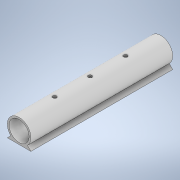
# Autodesk Inventor part: Cylinder
Saved by Autodesk Inventor 2022 (Build 260153000, 153)
## iProperties
Created: 2022-02-25
Part Number: Cylinder
Material: Generic
Document SubType Name: Modeling
Designer: Alexa
Density: 1 g/cm^3
Appearance: Default
Author: Alexa
Autodesk Inventor part; units mm, degrees
ref_plane "YZ Plane" through (0, 0, 0) normal (1, 0, 0) x (0, 1, 0)
ref_plane "XZ Plane" through (0, 0, 0) normal (0, 1, 0) x (-1, 0, 0)
ref_plane "XY Plane" through (0, 0, 0) normal (0, 0, 1) x (1, 0, 0)
sketch "Sketch1" plane through (0, 0, 0) normal (0, 1, 0) x (-1, 0, 0)
  line L0 (0, 0) -> (20, 0)
  line L1 (20, 0) -> (20, -120)
  line L2 (20, -120) -> (0, -120)
  line L3 (0, -120) -> (0, 0)
  dimension "d0" = 20
  dimension "d1" = 120
  constraints: 8 end point, 2 parallel, 1 horizontal, 1 perpendicular
  measures "d0" distance of L1.end L2.end
  measures "d1" distance of L0.end L1.end
extrude "Extrusion1" add sketch "Sketch1" along normal blind 20
sketch "Sketch2" plane through (0, 20, 0) normal (0, 1, 0) x (1, 0, 0)
  line L0 (-20, 120) -> (-20, 0) projected
  line L1 (0, 0) -> (0, 120) projected
  line L2 (-20, 0) -> (0, 0)
  line L3 (0, 0) -> (0, 120)
  line L4 (0, 120) -> (-20, 120)
  line L5 (-20, 120) -> (-20, 0)
  line L6 (0, 120) -> (-20, 120) projected
  line L7 (-20, 0) -> (-10, 0)
  line L8 (-10, 0) -> (-10, 120)
  line L9 (-10, 120) -> (-20, 120)
  line L10 (-20, 120) -> (-20, 0)
  line L11 (-10, 0) -> (-10, 60)
  line L12 (-10, 60) -> (-10, 90)
  line L13 (-10, 90) -> (-10, 30)
  circle A0 centre (-10, 30) radius 1.6
  circle A1 centre (-10, 60) radius 1.6
  circle A2 centre (-10, 90) radius 1.6
  dimension "d23" = 0
  dimension "d4" = 60
  dimension "d5" = 30
  dimension "d6" = 60
  dimension "d7" = 3.2
  dimension "d8" = 3.2
  dimension "d9" = 3.2
  constraints: 22 end point, 4 parallel, 3 centre point, 3 coincident, 3 midpoint, 2 horizontal, 2 perpendicular, 1 point on line
  measures "d4" distance of L7.end L11.end
  measures "d5" distance of L11.end L12.end
  measures "d6" distance of L12.end L13.end
  measures "d7" diameter of A0
  measures "d8" diameter of A1
  measures "d9" diameter of A2
extrude "Extrusion2" cut sketch "Sketch2" against normal blind 35.5625 contours A2 L8 | L8 A2 | A0 L8 | L8 A0 | A1 L8 | L8 A1
sketch "Sketch3" plane through (-20, 0, 0) normal (0, 0, 1) x (1, 0, 0)
  line L0 (0, 20) -> (20, 20) projected
  line L1 (0, 20) -> (20, 0)
  line L2 (20, 0) -> (20, 20)
  line L3 (0, 0) -> (20, 0) projected
  line L4 (20, 20) -> (0, 0)
  circle A0 centre (10, 10) radius 10
  line L5 (0, 0) -> (20, 0)
  line L6 (20, 0) -> (20, -2)
  line L7 (20, -2) -> (0, -2)
  line L8 (0, -2) -> (0, 0)
  line L9 (0, 0) -> (0, 20) projected
  line L10 (0, 20) -> (20, 20)
  line L11 (20, 20) -> (20, 0)
  line L12 (20, 0) -> (0, 0)
  line L13 (0, 0) -> (0, 20)
  point P0 (0, 10)
  point P1 (2.9289, 2.9289)
  point P2 (10, 20)
  point P3 (20, 10)
  point P4 (17.0711, 2.9289)
  dimension "d12" = 2
  constraints: 22 end point, 4 parallel, 4 perpendicular, 2 horizontal, 1 centre point, 1 midpoint, 1 tangent
  measures "d12" distance of L5.end L6.end
extrude "Extrusion3" cut sketch "Sketch3" against normal blind 223.2 contours L0 A0 L1 | L1 A0 L9 | L0 L4 A0 | A0 L4 L9 | L2 A0 L4 | L2 L1 A0
sketch "Sketch4" plane through (-20, 0, 0) normal (0, 0, 1) x (1, 0, 0)
  arc A0 (17.0711, 2.9289) -> (2.9289, 2.9289) centre (10, 10) ccw projected
  circle A1 centre (10, 10) radius 10
  circle A2 centre (10, 10) radius 8.5
  point P0 (20, 0)
  dimension "d15" = 17
  constraints: 2 centre point, 2 coincident
  measures "d15" diameter of A2
extrude "Extrusion4" cut sketch "Sketch4" against normal blind 267.3375 contours A2
sketch "Sketch6" plane through (0, 0, 0) normal (0, -1, 0) x (1, 0, 0)
  circle A0 centre (-10, -30) radius 1.6 projected
  circle A1 centre (-10, -30) radius 1.6
  circle A2 centre (-10, -60) radius 1.6 projected
  circle A3 centre (-10, -60) radius 1.6
  circle A4 centre (-10, -90) radius 1.6 projected
  circle A5 centre (-10, -90) radius 1.6
  point P0 (0, 0)
  constraints: 3 centre point, 3 coincident
extrude "Extrusion6" add sketch "Sketch6" against normal blind 3
sketch "Sketch7" plane through (-20, 0, 0) normal (0, 0, 1) x (1, 0, 0)
  circle A0 centre (10, 10) radius 8.5 projected
  circle A1 centre (10, 10) radius 8.5
  point P0 (20, 0)
  constraints: 1 centre point, 1 coincident
extrude "Extrusion7" add sketch "Sketch7" against normal blind 120
sketch "Sketch8" plane through (-20, 0, 0) normal (0, 0, 1) x (1, 0, 0)
  arc A0 (17.0711, 2.9289) -> (2.9289, 2.9289) centre (10, 10) ccw projected
  circle A1 centre (10, 10) radius 8.5
  point P0 (20, 0)
  dimension "d24" = 17
  constraints: 1 centre point, 1 coincident
  measures "d24" diameter of A1
extrude "Extrusion8" cut sketch "Sketch8" against normal blind 241.95
body "Solid1"
